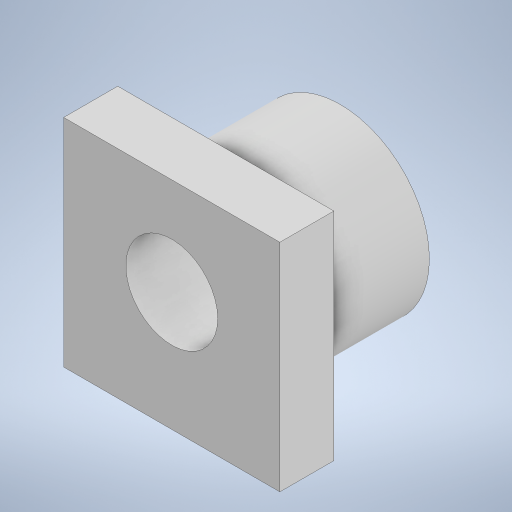
# Autodesk Inventor part: Cam
Saved by Autodesk Inventor 2023.1 (Build 271208000, 208)
## iProperties
Created: 2022-10-29
Part Number: Cam
Material: Generic
Document SubType Name: Modeling
Designer: nicol
Density: 1 g/cm^3
Appearance: Default
Author: nicol
Autodesk Inventor part; units mm, degrees
ref_plane "YZ Plane" through (0, 0, 0) normal (1, 0, 0) x (0, 1, 0)
ref_plane "XZ Plane" through (0, 0, 0) normal (0, 1, 0) x (-1, 0, 0)
ref_plane "XY Plane" through (0, 0, 0) normal (0, 0, 1) x (1, 0, 0)
sketch "Sketch1" plane through (0, 0, 0) normal (0, 0, 1) x (1, 0, 0)
  circle A0 centre (0, 0.6) radius 2.55
  circle A1 centre (0, 0) radius 4.95
  circle A2 centre (0, 0.6) radius 4.35 construction
  point P0 (-2.2057, -0.6796)
  dimension "d0" = 5.1
  dimension "d1" = 1.8
  dimension "d7" = 9.9
  constraints: 2 centre point, 1 coincident, 1 tangent, 1 vertical alignment, 3 other
  measures "d7" diameter of A1
extrude "Extrusion1" add sketch "Sketch1" along normal blind 6.35
sketch "Sketch2" plane through (0, 0, 6.35) normal (0, 0, 1) x (1, 0, 0)
  line L0 (-6, 6) -> (6, 6)
  line L1 (6, 6) -> (6, -6)
  line L2 (6, -6) -> (-6, -6)
  line L3 (-6, -6) -> (-6, 6)
  line L4 (6, 6) -> (-6, -6) construction
  circle A0 centre (0, 0) radius 4.95 projected
  circle A1 centre (0, 0.6) radius 2.55 projected
  dimension "d4" = 12
  constraints: 10 end point, 2 parallel, 2 perpendicular, 1 coincident, 1 horizontal, 1 midpoint
  measures "d4" distance of L0.start L0.end
extrude "Extrusion2" add sketch "Sketch2" along normal blind 3 contours L0 L1 L2 L3 | A0
body "Solid1"
